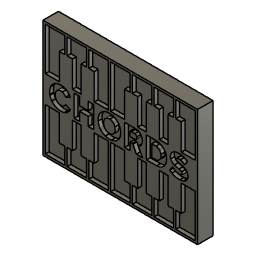
CHORDS Token (Autodesk Fusion 360 design; units mm, degrees)
Autodesk Fusion 360 part; units mm, degrees
(part 1 of 2)
sketch "Sketch1" plane through (0, 0, 0) normal (0, 0, 1) x (1, 0, 0)
  spline S0 degree 3 poles (0.0228, -10.5702) (0.0228, -7.0468) (0.0228, -3.5348) (0.0228, -0.0228) knots 0 0 0 0 1 1 1 1
  spline S1 degree 3 poles (0.0228, -0.0228) (13.3419, -0.0228) (26.6609, -0.0228) (39.98, -0.0228) knots 0 0 0 0 1 1 1 1
  spline S2 degree 3 poles (39.98, -0.0228) (39.98, -10.107) (39.98, -20.1912) (39.98, -30.2754) knots 0 0 0 0 1 1 1 1
  spline S3 degree 3 poles (39.98, -30.2754) (26.6609, -30.2754) (13.3419, -30.2754) (0.0228, -30.2754) knots 0 0 0 0 1 1 1 1
  spline S4 degree 3 poles (0.0228, -30.2754) (0.0228, -23.7108) (0.0228, -17.1462) (0.0228, -10.5702) knots 0 0 0 0 1 1 1 1
  spline S5 degree 3 poles (1.4466, -0.5923) (1.1634, -0.5923) (0.8802, -0.5923) (0.5988, -0.5923) knots 0 0 0 0 1 1 1 1
  spline S6 degree 3 poles (0.5988, -0.5923) (0.5988, -4.2974) (0.5988, -7.9893) (0.5988, -11.68) knots 0 0 0 0 1 1 1 1
  spline S7 degree 3 poles (0.5988, -11.68) (1.8142, -11.68) (3.0232, -11.68) (4.2411, -11.68) knots 0 0 0 0 1 1 1 1
  spline S8 degree 3 poles (4.2411, -11.68) (4.2411, -9.409) (4.2411, -7.1446) (4.2411, -4.8711) knots 0 0 0 0 1 1 1 1
  spline S9 degree 3 poles (4.2411, -4.8711) (4.715, -4.8711) (5.1799, -4.8711) (5.643, -4.8711) knots 0 0 0 0 1 1 1 1
  spline S10 degree 3 poles (5.643, -4.8711) (5.643, -3.4404) (5.643, -2.0188) (5.643, -0.5923) knots 0 0 0 0 1 1 1 1
  spline S11 degree 3 poles (5.643, -0.5923) (4.2474, -0.5923) (2.8584, -0.5923) (1.4466, -0.5923) knots 0 0 0 0 1 1 1 1
  spline S12 degree 3 poles (35.7656, -24.9334) (35.7656, -25.0951) (35.7656, -25.2569) (35.7656, -25.4274) knots 0 0 0 0 1 1 1 1
  spline S13 degree 3 poles (35.7656, -25.4274) (35.2876, -25.4274) (34.8227, -25.4274) (34.3599, -25.4274) knots 0 0 0 0 1 1 1 1
  spline S14 degree 3 poles (34.3599, -25.4274) (34.3599, -26.8581) (34.3599, -28.2796) (34.3599, -29.6993) knots 0 0 0 0 1 1 1 1
  spline S15 degree 3 poles (34.3599, -29.6993) (36.0463, -29.6993) (37.726, -29.6993) (39.4039, -29.6993) knots 0 0 0 0 1 1 1 1
  spline S16 degree 3 poles (39.4039, -29.6993) (39.4039, -26.0006) (39.4039, -22.3087) (39.4039, -18.6184) knots 0 0 0 0 1 1 1 1
  spline S17 degree 3 poles (39.4039, -18.6184) (38.1884, -18.6184) (36.9794, -18.6184) (35.7656, -18.6184) knots 0 0 0 0 1 1 1 1
  spline S18 degree 3 poles (35.7656, -18.6184) (35.7656, -20.7202) (35.7656, -22.8154) (35.7656, -24.9334) knots 0 0 0 0 1 1 1 1
  spline S19 degree 3 poles (18.0992, -18.6118) (17.8919, -18.6118) (17.6847, -18.6118) (17.4792, -18.6118) knots 0 0 0 0 1 1 1 1
  spline S20 degree 3 poles (17.4792, -18.6118) (17.4792, -22.3169) (17.4792, -26.0088) (17.4792, -29.6995) knots 0 0 0 0 1 1 1 1
  spline S21 degree 3 poles (17.4792, -29.6995) (19.1654, -29.6995) (20.8452, -29.6995) (22.5235, -29.6995) knots 0 0 0 0 1 1 1 1
  spline S22 degree 3 poles (22.5235, -29.6995) (22.5235, -28.2714) (22.5235, -26.8498) (22.5235, -25.4192) knots 0 0 0 0 1 1 1 1
  spline S23 degree 3 poles (22.5235, -25.4192) (22.0522, -25.4192) (21.5873, -25.4192) (21.1136, -25.4192) knots 0 0 0 0 1 1 1 1
  spline S24 degree 3 poles (21.1136, -25.4192) (21.1136, -23.1456) (21.1136, -20.8812) (21.1136, -18.6118) knots 0 0 0 0 1 1 1 1
  spline S25 degree 3 poles (21.1136, -18.6118) (20.1104, -18.6118) (19.1162, -18.6118) (18.0992, -18.6118) knots 0 0 0 0 1 1 1 1
  spline S26 degree 3 poles (13.2014, -29.7059) (14.4337, -29.7059) (15.6659, -29.7059) (16.8968, -29.7059) knots 0 0 0 0 1 1 1 1
  spline S27 degree 3 poles (16.8968, -29.7059) (16.8968, -26.0009) (16.8968, -22.309) (16.8968, -18.6182) knots 0 0 0 0 1 1 1 1
  spline S28 degree 3 poles (16.8968, -18.6182) (15.6814, -18.6182) (14.4725, -18.6182) (13.2545, -18.6182) knots 0 0 0 0 1 1 1 1
  spline S29 degree 3 poles (13.2545, -18.6182) (13.2545, -20.8891) (13.2545, -23.1535) (13.2545, -25.427) knots 0 0 0 0 1 1 1 1
  spline S30 degree 3 poles (13.2545, -25.427) (12.7807, -25.427) (12.3158, -25.427) (11.8524, -25.427) knots 0 0 0 0 1 1 1 1
  spline S31 degree 3 poles (11.8524, -25.427) (11.8524, -26.8577) (11.8524, -28.2793) (11.8524, -29.7059) knots 0 0 0 0 1 1 1 1
  spline S32 degree 3 poles (11.8524, -29.7059) (12.2988, -29.7059) (12.7387, -29.7059) (13.2014, -29.7059) knots 0 0 0 0 1 1 1 1
  spline S33 degree 3 poles (0.5923, -23.5438) (0.5923, -25.5961) (0.5923, -27.6485) (0.5923, -29.6995) knots 0 0 0 0 1 1 1 1
  spline S34 degree 3 poles (0.5923, -29.6995) (2.285, -29.6995) (3.9647, -29.6995) (5.6431, -29.6995) knots 0 0 0 0 1 1 1 1
  spline S35 degree 3 poles (5.6431, -29.6995) (5.6431, -28.2714) (5.6431, -26.8498) (5.6431, -25.4192) knots 0 0 0 0 1 1 1 1
  spline S36 degree 3 poles (5.6431, -25.4192) (5.1718, -25.4192) (4.7069, -25.4192) (4.2331, -25.4192) knots 0 0 0 0 1 1 1 1
  spline S37 degree 3 poles (4.2331, -25.4192) (4.2331, -23.1456) (4.2331, -20.8812) (4.2331, -18.6184) knots 0 0 0 0 1 1 1 1
  spline S38 degree 3 poles (4.2331, -18.6184) (3.0151, -18.6184) (1.8062, -18.6184) (0.5923, -18.6184) knots 0 0 0 0 1 1 1 1
  spline S39 degree 3 poles (0.5923, -18.6184) (0.5923, -20.2569) (0.5923, -21.889) (0.5923, -23.5438) knots 0 0 0 0 1 1 1 1
  spline S40 degree 3 poles (39.4105, -11.5811) (39.4105, -7.9193) (39.4105, -4.2574) (39.4105, -0.5998) knots 0 0 0 0 1 1 1 1
  spline S41 degree 3 poles (39.4105, -0.5998) (37.7158, -0.5998) (36.036, -0.5998) (34.3607, -0.5998) knots 0 0 0 0 1 1 1 1
  spline S42 degree 3 poles (34.3607, -0.5998) (34.3607, -2.0289) (34.3607, -3.4505) (34.3607, -4.8812) knots 0 0 0 0 1 1 1 1
  spline S43 degree 3 poles (34.3607, -4.8812) (34.8331, -4.8812) (35.2981, -4.8812) (35.7718, -4.8812) knots 0 0 0 0 1 1 1 1
  spline S44 degree 3 poles (35.7718, -4.8812) (35.7718, -7.1548) (35.7718, -9.4192) (35.7718, -11.6865) knots 0 0 0 0 1 1 1 1
  spline S45 degree 3 poles (35.7718, -11.6865) (36.9652, -11.6865) (38.1496, -11.6858) (39.3339, -11.6881) knots 0 0 0 0 1 1 1 1
  spline S46 degree 3 poles (39.3339, -11.6881) (39.4036, -11.6882) (39.4194, -11.6627) (39.4105, -11.5811) knots 0 0 0 0 1 1 1 1
  spline S47 degree 3 poles (16.9032, -10.2855) (16.9032, -7.0562) (16.9032, -3.8269) (16.9032, -0.5987) knots 0 0 0 0 1 1 1 1
  spline S48 degree 3 poles (16.9032, -0.5987) (15.2107, -0.5987) (13.5309, -0.5987) (11.8524, -0.5987) knots 0 0 0 0 1 1 1 1
  spline S49 degree 3 poles (11.8524, -0.5987) (11.8524, -2.0267) (11.8524, -3.4483) (11.8524, -4.8789) knots 0 0 0 0 1 1 1 1
  spline S50 degree 3 poles (11.8524, -4.8789) (12.3236, -4.8789) (12.7885, -4.8789) (13.2623, -4.8789) knots 0 0 0 0 1 1 1 1
  spline S51 degree 3 poles (13.2623, -4.8789) (13.2623, -7.1525) (13.2623, -9.4169) (13.2623, -11.6799) knots 0 0 0 0 1 1 1 1
  spline S52 degree 3 poles (13.2623, -11.6799) (14.4802, -11.6799) (15.6892, -11.6799) (16.9032, -11.6799) knots 0 0 0 0 1 1 1 1
  spline S53 degree 3 poles (16.9032, -11.6799) (16.9032, -11.2184) (16.9032, -10.7633) (16.9032, -10.2855) knots 0 0 0 0 1 1 1 1
  spline S54 degree 3 poles (21.1176, -8.1213) (21.1176, -7.0409) (21.1176, -5.9605) (21.1176, -4.871) knots 0 0 0 0 1 1 1 1
  spline S55 degree 3 poles (21.1176, -4.871) (21.5955, -4.871) (22.0604, -4.871) (22.5234, -4.871) knots 0 0 0 0 1 1 1 1
  spline S56 degree 3 poles (22.5234, -4.871) (22.5234, -3.4403) (22.5234, -2.0187) (22.5234, -0.5989) knots 0 0 0 0 1 1 1 1
  spline S57 degree 3 poles (22.5234, -0.5989) (20.8371, -0.5989) (19.1573, -0.5989) (17.4793, -0.5989) knots 0 0 0 0 1 1 1 1
  spline S58 degree 3 poles (17.4793, -0.5989) (17.4793, -4.2975) (17.4793, -7.9895) (17.4793, -11.6799) knots 0 0 0 0 1 1 1 1
  spline S59 degree 3 poles (17.4793, -11.6799) (18.6947, -11.6799) (19.9037, -11.6799) (21.1176, -11.6799) knots 0 0 0 0 1 1 1 1
  spline S60 degree 3 poles (21.1176, -11.6799) (21.1176, -10.4969) (21.1176, -9.3205) (21.1176, -8.1213) knots 0 0 0 0 1 1 1 1
  spline S61 degree 3 poles (11.2764, -0.6533) (11.2844, -0.5523) (11.2065, -0.5941) (11.1663, -0.5941) knots 0 0 0 0 1 1 1 1
  spline S62 degree 3 poles (11.1663, -0.5941) (9.549, -0.592) (7.9316, -0.5923) (6.3143, -0.5923) knots 0 0 0 0 1 1 1 1
  spline S63 degree 3 poles (6.3143, -0.5923) (6.2851, -0.5923) (6.2559, -0.5923) (6.2243, -0.5923) knots 0 0 0 0 1 1 1 1
  spline S64 degree 3 poles (6.2243, -0.5923) (6.2243, -2.0242) (6.2243, -3.4458) (6.2243, -4.8764) knots 0 0 0 0 1 1 1 1
  spline S65 degree 3 poles (6.2243, -4.8764) (6.6943, -4.8764) (7.1592, -4.8764) (7.633, -4.8764) knots 0 0 0 0 1 1 1 1
  spline S66 degree 3 poles (7.633, -4.8764) (7.633, -7.15) (7.633, -9.4144) (7.633, -11.6812) knots 0 0 0 0 1 1 1 1
  spline S67 degree 3 poles (7.633, -11.6812) (8.3802, -11.6812) (9.1183, -11.6812) (9.8655, -11.6812) knots 0 0 0 0 1 1 1 1
  spline S68 degree 3 poles (9.8655, -11.6812) (9.8655, -9.4115) (9.8655, -7.147) (9.8655, -4.8735) knots 0 0 0 0 1 1 1 1
  spline S69 degree 3 poles (9.8655, -4.8735) (10.3393, -4.8735) (10.8042, -4.8735) (11.2764, -4.8735) knots 0 0 0 0 1 1 1 1
  spline S70 degree 3 poles (11.2764, -4.8735) (11.2764, -3.4681) (11.2764, -2.0718) (11.2764, -0.6533) knots 0 0 0 0 1 1 1 1
  spline S71 degree 3 poles (30.5374, -29.7059) (31.6178, -29.7059) (32.6982, -29.7059) (33.7772, -29.7059) knots 0 0 0 0 1 1 1 1
  spline S72 degree 3 poles (33.7772, -29.7059) (33.7772, -28.2714) (33.7772, -26.8498) (33.7772, -25.4192) knots 0 0 0 0 1 1 1 1
  spline S73 degree 3 poles (33.7772, -25.4192) (33.3058, -25.4192) (32.8409, -25.4192) (32.3672, -25.4192) knots 0 0 0 0 1 1 1 1
  spline S74 degree 3 poles (32.3672, -25.4192) (32.3672, -23.1457) (32.3672, -20.8813) (32.3672, -18.6183) knots 0 0 0 0 1 1 1 1
  spline S75 degree 3 poles (32.3672, -18.6183) (31.6201, -18.6183) (30.8819, -18.6183) (30.1348, -18.6183) knots 0 0 0 0 1 1 1 1
  spline S76 degree 3 poles (30.1348, -18.6183) (30.1348, -20.8893) (30.1348, -23.1537) (30.1348, -25.4271) knots 0 0 0 0 1 1 1 1
  spline S77 degree 3 poles (30.1348, -25.4271) (29.661, -25.4271) (29.1961, -25.4271) (28.7329, -25.4271) knots 0 0 0 0 1 1 1 1
  spline S78 degree 3 poles (28.7329, -25.4271) (28.7329, -26.8578) (28.7329, -28.2794) (28.7329, -29.7059) knots 0 0 0 0 1 1 1 1
  spline S79 degree 3 poles (28.7329, -29.7059) (29.3312, -29.7059) (29.9229, -29.7059) (30.5374, -29.7059) knots 0 0 0 0 1 1 1 1
  spline S80 degree 3 poles (26.0952, -29.7059) (26.7808, -29.7059) (27.4663, -29.7059) (28.1503, -29.7059) knots 0 0 0 0 1 1 1 1
  spline S81 degree 3 poles (28.1503, -29.7059) (28.1503, -28.2713) (28.1503, -26.8497) (28.1503, -25.4191) knots 0 0 0 0 1 1 1 1
  spline S82 degree 3 poles (28.1503, -25.4191) (27.679, -25.4191) (27.2141, -25.4191) (26.7404, -25.4191) knots 0 0 0 0 1 1 1 1
  spline S83 degree 3 poles (26.7404, -25.4191) (26.7404, -23.1456) (26.7404, -20.8812) (26.7404, -18.6183) knots 0 0 0 0 1 1 1 1
  spline S84 degree 3 poles (26.7404, -18.6183) (25.9932, -18.6183) (25.255, -18.6183) (24.5079, -18.6183) knots 0 0 0 0 1 1 1 1
  spline S85 degree 3 poles (24.5079, -18.6183) (24.5079, -20.8893) (24.5079, -23.1537) (24.5079, -25.4272) knots 0 0 0 0 1 1 1 1
  spline S86 degree 3 poles (24.5079, -25.4272) (24.0341, -25.4272) (23.5692, -25.4272) (23.1061, -25.4272) knots 0 0 0 0 1 1 1 1
  spline S87 degree 3 poles (23.1061, -25.4272) (23.1061, -26.8579) (23.1061, -28.2794) (23.1061, -29.7059) knots 0 0 0 0 1 1 1 1
  spline S88 degree 3 poles (23.1061, -29.7059) (24.0993, -29.7059) (25.0858, -29.7059) (26.0952, -29.7059) knots 0 0 0 0 1 1 1 1
  spline S89 degree 3 poles (11.2764, -29.1478) (11.2764, -27.908) (11.2764, -26.6681) (11.2764, -25.4192) knots 0 0 0 0 1 1 1 1
  spline S90 degree 3 poles (11.2764, -25.4192) (10.7986, -25.4192) (10.3337, -25.4192) (9.86, -25.4192) knots 0 0 0 0 1 1 1 1
  spline S91 degree 3 poles (9.86, -25.4192) (9.86, -23.1457) (9.86, -20.8813) (9.86, -18.6183) knots 0 0 0 0 1 1 1 1
  spline S92 degree 3 poles (9.86, -18.6183) (9.1128, -18.6183) (8.3747, -18.6183) (7.6276, -18.6183) knots 0 0 0 0 1 1 1 1
  spline S93 degree 3 poles (7.6276, -18.6183) (7.6276, -20.8892) (7.6276, -23.1536) (7.6276, -25.4271) knots 0 0 0 0 1 1 1 1
  spline S94 degree 3 poles (7.6276, -25.4271) (7.1538, -25.4271) (6.6889, -25.4271) (6.2256, -25.4271) knots 0 0 0 0 1 1 1 1
  spline S95 degree 3 poles (6.2256, -25.4271) (6.2256, -26.8578) (6.2256, -28.2793) (6.2256, -29.6994) knots 0 0 0 0 1 1 1 1
  spline S96 degree 3 poles (6.2256, -29.6994) (7.9119, -29.6994) (9.5916, -29.6994) (11.2764, -29.6994) knots 0 0 0 0 1 1 1 1
  spline S97 degree 3 poles (11.2764, -29.6994) (11.2764, -29.5188) (11.2764, -29.3447) (11.2764, -29.1478) knots 0 0 0 0 1 1 1 1
  spline S98 degree 3 poles (30.1388, -7.9618) (30.1388, -9.2017) (30.1388, -10.4415) (30.1388, -11.6799) knots 0 0 0 0 1 1 1 1
  spline S99 degree 3 poles (30.1388, -11.6799) (30.8899, -11.6799) (31.6281, -11.6799) (32.3752, -11.6799) knots 0 0 0 0 1 1 1 1
  spline S100 degree 3 poles (32.3752, -11.6799) (32.3752, -9.409) (32.3752, -7.1446) (32.3752, -4.8711) knots 0 0 0 0 1 1 1 1
  spline S101 degree 3 poles (32.3752, -4.8711) (32.849, -4.8711) (33.3139, -4.8711) (33.7771, -4.8711) knots 0 0 0 0 1 1 1 1
  spline S102 degree 3 poles (33.7771, -4.8711) (33.7771, -3.4404) (33.7771, -2.0189) (33.7771, -0.5988) knots 0 0 0 0 1 1 1 1
  spline S103 degree 3 poles (33.7771, -0.5988) (32.0909, -0.5988) (30.4112, -0.5988) (28.7329, -0.5988) knots 0 0 0 0 1 1 1 1
  spline S104 degree 3 poles (28.7329, -0.5988) (28.7329, -2.0269) (28.7329, -3.4484) (28.7329, -4.8791) knots 0 0 0 0 1 1 1 1
  spline S105 degree 3 poles (28.7329, -4.8791) (29.2042, -4.8791) (29.6691, -4.8791) (30.1388, -4.8791) knots 0 0 0 0 1 1 1 1
  spline S106 degree 3 poles (30.1388, -4.8791) (30.1388, -5.9051) (30.1388, -6.9221) (30.1388, -7.9618) knots 0 0 0 0 1 1 1 1
  spline S107 degree 3 poles (26.7445, -9.4198) (26.7445, -7.9066) (26.7445, -6.3934) (26.7445, -4.8711) knots 0 0 0 0 1 1 1 1
  spline S108 degree 3 poles (26.7445, -4.8711) (27.2222, -4.8711) (27.6871, -4.8711) (28.1503, -4.8711) knots 0 0 0 0 1 1 1 1
  spline S109 degree 3 poles (28.1503, -4.8711) (28.1503, -3.4404) (28.1503, -2.0189) (28.1503, -0.5988) knots 0 0 0 0 1 1 1 1
  spline S110 degree 3 poles (28.1503, -0.5988) (26.4641, -0.5988) (24.7843, -0.5988) (23.1061, -0.5988) knots 0 0 0 0 1 1 1 1
  spline S111 degree 3 poles (23.1061, -0.5988) (23.1061, -2.0269) (23.1061, -3.4484) (23.1061, -4.8791) knots 0 0 0 0 1 1 1 1
  spline S112 degree 3 poles (23.1061, -4.8791) (23.5774, -4.8791) (24.0423, -4.8791) (24.516, -4.8791) knots 0 0 0 0 1 1 1 1
  spline S113 degree 3 poles (24.516, -4.8791) (24.516, -7.1526) (24.516, -9.417) (24.516, -11.6799) knots 0 0 0 0 1 1 1 1
  spline S114 degree 3 poles (24.516, -11.6799) (25.2631, -11.6799) (26.0013, -11.6799) (26.7445, -11.6799) knots 0 0 0 0 1 1 1 1
  spline S115 degree 3 poles (26.7445, -11.6799) (26.7445, -10.9298) (26.7445, -10.1862) (26.7445, -9.4198) knots 0 0 0 0 1 1 1 1
  spline S116 degree 3 poles (31.2674, -17.0863) (31.401, -16.8984) (31.5593, -16.7233) (31.6638, -16.5205) knots 0 0 0 0 1 1 1 1
  spline S117 degree 3 poles (31.6638, -16.5205) (32.0308, -15.8079) (32.0758, -15.0551) (31.8752, -14.2875) knots 0 0 0 0 1 1 1 1
  spline S118 degree 3 poles (31.8752, -14.2875) (31.68, -13.5405) (31.2249, -12.9974) (30.5351, -12.6532) knots 0 0 0 0 1 1 1 1
  spline S119 degree 3 poles (30.5351, -12.6532) (30.0644, -12.4183) (29.5596, -12.329) (29.0381, -12.3269) knots 0 0 0 0 1 1 1 1
  spline S120 degree 3 poles (29.0381, -12.3269) (28.3054, -12.3239) (27.5727, -12.3261) (26.8399, -12.3261) knots 0 0 0 0 1 1 1 1
  spline S121 degree 3 poles (26.8399, -12.3261) (26.8108, -12.3261) (26.7817, -12.3261) (26.7518, -12.3261) knots 0 0 0 0 1 1 1 1
  spline S122 degree 3 poles (26.7518, -12.3261) (26.7518, -14.2063) (26.7518, -16.0754) (26.7518, -17.9291) knots 0 0 0 0 1 1 1 1
  spline S123 degree 3 poles (26.7518, -17.9291) (27.6506, -17.9291) (28.5433, -17.9582) (29.4331, -17.9199) knots 0 0 0 0 1 1 1 1
  spline S124 degree 3 poles (29.4331, -17.9199) (30.1342, -17.8896) (30.7554, -17.6092) (31.2674, -17.0863) knots 0 0 0 0 1 1 1 1
  spline S125 degree 3 poles (25.0567, -12.7014) (24.6935, -12.4266) (24.2757, -12.3262) (23.8296, -12.325) knots 0 0 0 0 1 1 1 1
  spline S126 degree 3 poles (23.8296, -12.325) (22.9565, -12.3226) (22.0835, -12.3243) (21.2104, -12.3245) knots 0 0 0 0 1 1 1 1
  spline S127 degree 3 poles (21.2104, -12.3245) (21.1813, -12.3245) (21.1523, -12.327) (21.1233, -12.3284) knots 0 0 0 0 1 1 1 1
  spline S128 degree 3 poles (21.1233, -12.3284) (21.1233, -14.2057) (21.1233, -16.0751) (21.1233, -17.9455) knots 0 0 0 0 1 1 1 1
  spline S129 degree 3 poles (21.1233, -17.9455) (21.5938, -17.9455) (22.0586, -17.9455) (22.5324, -17.9455) knots 0 0 0 0 1 1 1 1
  spline S130 degree 3 poles (22.5324, -17.9455) (22.5324, -17.308) (22.5324, -16.6761) (22.5324, -16.0376) knots 0 0 0 0 1 1 1 1
  spline S131 degree 3 poles (22.5324, -16.0376) (22.7418, -16.0376) (22.9424, -16.0425) (23.1426, -16.0352) knots 0 0 0 0 1 1 1 1
  spline S132 degree 3 poles (23.1426, -16.0352) (23.2246, -16.0322) (23.2595, -16.0634) (23.2923, -16.1331) knots 0 0 0 0 1 1 1 1
  spline S133 degree 3 poles (23.2923, -16.1331) (23.5772, -16.739) (23.866, -17.3431) (24.1535, -17.9475) knots 0 0 0 0 1 1 1 1
  spline S134 degree 3 poles (24.1535, -17.9475) (24.6869, -17.9475) (25.2172, -17.9475) (25.7624, -17.9475) knots 0 0 0 0 1 1 1 1
  spline S135 degree 3 poles (25.7624, -17.9475) (25.39, -17.2541) (25.0223, -16.5698) (24.6542, -15.8845) knots 0 0 0 0 1 1 1 1
  spline S136 degree 3 poles (24.6542, -15.8845) (26.0292, -15.3556) (26.0221, -13.4204) (25.0567, -12.7014) knots 0 0 0 0 1 1 1 1
  spline S137 degree 3 poles (16.1529, -17.8935) (16.6625, -18.0645) (17.1838, -18.1067) (17.713, -18.02) knots 0 0 0 0 1 1 1 1
  spline S138 degree 3 poles (17.713, -18.02) (18.5444, -17.8837) (19.2139, -17.4852) (19.6675, -16.7638) knots 0 0 0 0 1 1 1 1
  spline S139 degree 3 poles (19.6675, -16.7638) (20.0864, -16.0975) (20.1938, -15.3643) (20.0663, -14.5989) knots 0 0 0 0 1 1 1 1
  spline S140 degree 3 poles (20.0663, -14.5989) (19.9233, -13.7403) (19.4853, -13.068) (18.7243, -12.6285) knots 0 0 0 0 1 1 1 1
  spline S141 degree 3 poles (18.7243, -12.6285) (18.1513, -12.2977) (17.5266, -12.1895) (16.8716, -12.2536) knots 0 0 0 0 1 1 1 1
  spline S142 degree 3 poles (16.8716, -12.2536) (16.0569, -12.3333) (15.3695, -12.6649) (14.8619, -13.3182) knots 0 0 0 0 1 1 1 1
  spline S143 degree 3 poles (14.8619, -13.3182) (14.3755, -13.9444) (14.2022, -14.6676) (14.2807, -15.4476) knots 0 0 0 0 1 1 1 1
  spline S144 degree 3 poles (14.2807, -15.4476) (14.4002, -16.6354) (15.0088, -17.4609) (16.1529, -17.8935) knots 0 0 0 0 1 1 1 1
  spline S145 degree 3 poles (10.6272, -14.4201) (10.2378, -14.4201) (9.8484, -14.4201) (9.4503, -14.4201) knots 0 0 0 0 1 1 1 1
  spline S146 degree 3 poles (9.4503, -14.4201) (9.4503, -13.7148) (9.4503, -13.0222) (9.4503, -12.3306) knots 0 0 0 0 1 1 1 1
  spline S147 degree 3 poles (9.4503, -12.3306) (8.9766, -12.3306) (8.5119, -12.3306) (8.0472, -12.3306) knots 0 0 0 0 1 1 1 1
  spline S148 degree 3 poles (8.0472, -12.3306) (8.0472, -14.206) (8.0472, -16.0752) (8.0472, -17.9455) knots 0 0 0 0 1 1 1 1
  spline S149 degree 3 poles (8.0472, -17.9455) (8.5177, -17.9455) (8.9824, -17.9455) (9.4552, -17.9455) knots 0 0 0 0 1 1 1 1
  spline S150 degree 3 poles (9.4552, -17.9455) (9.4552, -17.1901) (9.4552, -16.4402) (9.4552, -15.6849) knots 0 0 0 0 1 1 1 1
  spline S151 degree 3 poles (9.4552, -15.6849) (10.2088, -15.6849) (10.9543, -15.6849) (11.712, -15.6849) knots 0 0 0 0 1 1 1 1
  spline S152 degree 3 poles (11.712, -15.6849) (11.712, -16.4429) (11.712, -17.1955) (11.712, -17.9437) knots 0 0 0 0 1 1 1 1
  spline S153 degree 3 poles (11.712, -17.9437) (12.1889, -17.9437) (12.6537, -17.9437) (13.1148, -17.9437) knots 0 0 0 0 1 1 1 1
  spline S154 degree 3 poles (13.1148, -17.9437) (13.1148, -16.0672) (13.1148, -14.198) (13.1148, -12.3311) knots 0 0 0 0 1 1 1 1
  spline S155 degree 3 poles (13.1148, -12.3311) (12.6432, -12.3311) (12.1785, -12.3311) (11.7049, -12.3311) knots 0 0 0 0 1 1 1 1
  spline S156 degree 3 poles (11.7049, -12.3311) (11.7049, -13.0303) (11.7049, -13.7229) (11.7049, -14.4201) knots 0 0 0 0 1 1 1 1
  spline S157 degree 3 poles (11.7049, -14.4201) (11.3473, -14.4201) (10.9986, -14.4201) (10.6272, -14.4201) knots 0 0 0 0 1 1 1 1
  spline S158 degree 3 poles (35.429, -18.0595) (35.7152, -18.0078) (36.0122, -17.9886) (36.2859, -17.8987) knots 0 0 0 0 1 1 1 1
  spline S159 degree 3 poles (36.2859, -17.8987) (37.453, -17.5153) (37.6514, -16.4372) (37.4532, -15.7221) knots 0 0 0 0 1 1 1 1
  spline S160 degree 3 poles (37.4532, -15.7221) (37.3295, -15.2758) (37.0095, -15.0019) (36.6092, -14.8078) knots 0 0 0 0 1 1 1 1
  spline S161 degree 3 poles (36.6092, -14.8078) (36.1929, -14.6061) (35.7418, -14.5212) (35.2961, -14.416) knots 0 0 0 0 1 1 1 1
  spline S162 degree 3 poles (35.2961, -14.416) (35.0655, -14.3616) (34.8301, -14.3042) (34.6169, -14.2051) knots 0 0 0 0 1 1 1 1
  spline S163 degree 3 poles (34.6169, -14.2051) (34.3613, -14.0864) (34.3582, -13.7521) (34.5927, -13.5913) knots 0 0 0 0 1 1 1 1
  spline S164 degree 3 poles (34.5927, -13.5913) (34.6447, -13.5556) (34.7061, -13.5289) (34.7671, -13.5119) knots 0 0 0 0 1 1 1 1
  spline S165 degree 3 poles (34.7671, -13.5119) (35.019, -13.4418) (35.2713, -13.4707) (35.5216, -13.5236) knots 0 0 0 0 1 1 1 1
  spline S166 degree 3 poles (35.5216, -13.5236) (35.9294, -13.6098) (36.2925, -13.7907) (36.6186, -14.0557) knots 0 0 0 0 1 1 1 1
  spline S167 degree 3 poles (36.6186, -14.0557) (36.8759, -13.7079) (37.1302, -13.3644) (37.3871, -13.0172) knots 0 0 0 0 1 1 1 1
  spline S168 degree 3 poles (37.3871, -13.0172) (37.3229, -12.9656) (37.2652, -12.9163) (37.2046, -12.8709) knots 0 0 0 0 1 1 1 1
  spline S169 degree 3 poles (37.2046, -12.8709) (36.6315, -12.4423) (35.9773, -12.2575) (35.2711, -12.2358) knots 0 0 0 0 1 1 1 1
  spline S170 degree 3 poles (35.2711, -12.2358) (34.8576, -12.223) (34.4539, -12.2782) (34.0699, -12.4405) knots 0 0 0 0 1 1 1 1
  spline S171 degree 3 poles (34.0699, -12.4405) (33.2042, -12.8062) (32.7844, -13.6938) (33.074, -14.5448) knots 0 0 0 0 1 1 1 1
  spline S172 degree 3 poles (33.074, -14.5448) (33.2291, -15.0004) (33.5664, -15.2834) (33.9981, -15.4393) knots 0 0 0 0 1 1 1 1
  spline S173 degree 3 poles (33.9981, -15.4393) (34.3771, -15.5761) (34.7748, -15.6619) (35.1656, -15.765) knots 0 0 0 0 1 1 1 1
  spline S174 degree 3 poles (35.1656, -15.765) (35.4179, -15.8315) (35.6796, -15.8714) (35.9019, -16.0198) knots 0 0 0 0 1 1 1 1
  spline S175 degree 3 poles (35.9019, -16.0198) (36.1425, -16.1803) (36.1534, -16.4769) (35.9212, -16.649) knots 0 0 0 0 1 1 1 1
  spline S176 degree 3 poles (35.9212, -16.649) (35.8382, -16.7105) (35.7366, -16.7547) (35.6367, -16.784) knots 0 0 0 0 1 1 1 1
  spline S177 degree 3 poles (35.6367, -16.784) (35.4142, -16.8493) (35.1855, -16.8335) (34.9593, -16.8) knots 0 0 0 0 1 1 1 1
  spline S178 degree 3 poles (34.9593, -16.8) (34.416, -16.7195) (33.9548, -16.4754) (33.5594, -16.0811) knots 0 0 0 0 1 1 1 1
  spline S179 degree 3 poles (33.5594, -16.0811) (33.312, -16.4435) (33.0667, -16.8029) (32.8062, -17.1844) knots 0 0 0 0 1 1 1 1
  spline S180 degree 3 poles (32.8062, -17.1844) (32.9868, -17.3185) (33.1571, -17.4644) (33.3454, -17.5812) knots 0 0 0 0 1 1 1 1
  spline S181 degree 3 poles (33.3454, -17.5812) (33.9769, -17.9731) (34.6784, -18.0797) (35.429, -18.0595) knots 0 0 0 0 1 1 1 1
  spline S182 degree 3 poles (1.7635, -15.742) (1.8461, -16.1886) (2.0179, -16.5963) (2.2925, -16.9597) knots 0 0 0 0 1 1 1 1
  spline S183 degree 3 poles (2.2925, -16.9597) (3.0452, -17.956) (4.3949, -18.2671) (5.4961, -17.9369) knots 0 0 0 0 1 1 1 1
  spline S184 degree 3 poles (5.4961, -17.9369) (6.2227, -17.719) (6.7147, -17.2311) (7.0532, -16.5552) knots 0 0 0 0 1 1 1 1
  spline S185 degree 3 poles (7.0532, -16.5552) (6.6455, -16.3561) (6.2462, -16.1611) (5.8469, -15.9661) knots 0 0 0 0 1 1 1 1
  spline S186 degree 3 poles (5.8469, -15.9661) (5.6028, -16.4677) (5.2156, -16.7636) (4.6612, -16.7813) knots 0 0 0 0 1 1 1 1
  spline S187 degree 3 poles (4.6612, -16.7813) (4.104, -16.799) (3.665, -16.5497) (3.3893, -16.0671) knots 0 0 0 0 1 1 1 1
  spline S188 degree 3 poles (3.3893, -16.0671) (3.0431, -15.461) (3.0448, -14.8341) (3.3907, -14.2271) knots 0 0 0 0 1 1 1 1
  spline S189 degree 3 poles (3.3907, -14.2271) (3.7265, -13.6377) (4.4189, -13.3734) (5.0331, -13.581) knots 0 0 0 0 1 1 1 1
  spline S190 degree 3 poles (5.0331, -13.581) (5.4119, -13.709) (5.6784, -13.9656) (5.8446, -14.3334) knots 0 0 0 0 1 1 1 1
  spline S191 degree 3 poles (5.8446, -14.3334) (6.2483, -14.1361) (6.6476, -13.9409) (7.0529, -13.7428) knots 0 0 0 0 1 1 1 1
  spline S192 degree 3 poles (7.0529, -13.7428) (6.7834, -13.1999) (6.4138, -12.7708) (5.874, -12.507) knots 0 0 0 0 1 1 1 1
  spline S193 degree 3 poles (5.874, -12.507) (5.3126, -12.2327) (4.7174, -12.1777) (4.1098, -12.2797) knots 0 0 0 0 1 1 1 1
  spline S194 degree 3 poles (4.1098, -12.2797) (3.1324, -12.4438) (2.4019, -12.9553) (1.9794, -13.8657) knots 0 0 0 0 1 1 1 1
  spline S195 degree 3 poles (1.9794, -13.8657) (1.7044, -14.4582) (1.6566, -15.083) (1.7635, -15.742) knots 0 0 0 0 1 1 1 1
  spline S196 degree 3 poles (1.458, -0.5923) (2.8584, -0.5923) (4.2474, -0.5923) (5.643, -0.5923) knots 0 0 0 0 1 1 1 1
  spline S197 degree 3 poles (5.643, -0.5923) (5.643, -2.0188) (5.643, -3.4404) (5.643, -4.8711) knots 0 0 0 0 1 1 1 1
  spline S198 degree 3 poles (5.643, -4.8711) (5.1799, -4.8711) (4.715, -4.8711) (4.2411, -4.8711) knots 0 0 0 0 1 1 1 1
  spline S199 degree 3 poles (4.2411, -4.8711) (4.2411, -7.1446) (4.2411, -9.409) (4.2411, -11.68) knots 0 0 0 0 1 1 1 1
  spline S200 degree 3 poles (4.2411, -11.68) (3.0232, -11.68) (1.8142, -11.68) (0.5988, -11.68) knots 0 0 0 0 1 1 1 1
  spline S201 degree 3 poles (0.5988, -11.68) (0.5988, -7.9893) (0.5988, -4.2974) (0.5988, -0.5923) knots 0 0 0 0 1 1 1 1
  spline S202 degree 3 poles (0.5988, -0.5923) (0.8802, -0.5923) (1.1634, -0.5923) (1.458, -0.5923) knots 0 0 0 0 1 1 1 1
  spline S203 degree 3 poles (35.7656, -24.922) (35.7656, -22.8154) (35.7656, -20.7202) (35.7656, -18.6184) knots 0 0 0 0 1 1 1 1
  spline S204 degree 3 poles (35.7656, -18.6184) (36.9794, -18.6184) (38.1884, -18.6184) (39.4039, -18.6184) knots 0 0 0 0 1 1 1 1
  spline S205 degree 3 poles (39.4039, -18.6184) (39.4039, -22.3087) (39.4039, -26.0006) (39.4039, -29.6993) knots 0 0 0 0 1 1 1 1
  spline S206 degree 3 poles (39.4039, -29.6993) (37.726, -29.6993) (36.0463, -29.6993) (34.3599, -29.6993) knots 0 0 0 0 1 1 1 1
  spline S207 degree 3 poles (34.3599, -29.6993) (34.3599, -28.2796) (34.3599, -26.8581) (34.3599, -25.4274) knots 0 0 0 0 1 1 1 1
  spline S208 degree 3 poles (34.3599, -25.4274) (34.8227, -25.4274) (35.2876, -25.4274) (35.7656, -25.4274) knots 0 0 0 0 1 1 1 1
  spline S209 degree 3 poles (35.7656, -25.4274) (35.7656, -25.2569) (35.7656, -25.0951) (35.7656, -24.922) knots 0 0 0 0 1 1 1 1
  spline S210 degree 3 poles (18.1106, -18.6118) (19.1162, -18.6118) (20.1104, -18.6118) (21.1136, -18.6118) knots 0 0 0 0 1 1 1 1
  spline S211 degree 3 poles (21.1136, -18.6118) (21.1136, -20.8812) (21.1136, -23.1456) (21.1136, -25.4192) knots 0 0 0 0 1 1 1 1
  spline S212 degree 3 poles (21.1136, -25.4192) (21.5873, -25.4192) (22.0522, -25.4192) (22.5235, -25.4192) knots 0 0 0 0 1 1 1 1
  spline S213 degree 3 poles (22.5235, -25.4192) (22.5235, -26.8498) (22.5235, -28.2714) (22.5235, -29.6995) knots 0 0 0 0 1 1 1 1
  spline S214 degree 3 poles (22.5235, -29.6995) (20.8452, -29.6995) (19.1654, -29.6995) (17.4792, -29.6995) knots 0 0 0 0 1 1 1 1
  spline S215 degree 3 poles (17.4792, -29.6995) (17.4792, -26.0088) (17.4792, -22.3169) (17.4792, -18.6118) knots 0 0 0 0 1 1 1 1
  spline S216 degree 3 poles (17.4792, -18.6118) (17.6847, -18.6118) (17.8919, -18.6118) (18.1106, -18.6118) knots 0 0 0 0 1 1 1 1
  spline S217 degree 3 poles (13.19, -29.7059) (12.7387, -29.7059) (12.2988, -29.7059) (11.8524, -29.7059) knots 0 0 0 0 1 1 1 1
  spline S218 degree 3 poles (11.8524, -29.7059) (11.8524, -28.2793) (11.8524, -26.8577) (11.8524, -25.427) knots 0 0 0 0 1 1 1 1
  spline S219 degree 3 poles (11.8524, -25.427) (12.3158, -25.427) (12.7807, -25.427) (13.2545, -25.427) knots 0 0 0 0 1 1 1 1
  spline S220 degree 3 poles (13.2545, -25.427) (13.2545, -23.1535) (13.2545, -20.8891) (13.2545, -18.6182) knots 0 0 0 0 1 1 1 1
  spline S221 degree 3 poles (13.2545, -18.6182) (14.4725, -18.6182) (15.6814, -18.6182) (16.8968, -18.6182) knots 0 0 0 0 1 1 1 1
  spline S222 degree 3 poles (16.8968, -18.6182) (16.8968, -22.309) (16.8968, -26.0009) (16.8968, -29.7059) knots 0 0 0 0 1 1 1 1
  spline S223 degree 3 poles (16.8968, -29.7059) (15.6659, -29.7059) (14.4337, -29.7059) (13.19, -29.7059) knots 0 0 0 0 1 1 1 1
  spline S224 degree 3 poles (0.5923, -23.5324) (0.5923, -21.889) (0.5923, -20.2569) (0.5923, -18.6184) knots 0 0 0 0 1 1 1 1
  spline S225 degree 3 poles (0.5923, -18.6184) (1.8062, -18.6184) (3.0151, -18.6184) (4.2331, -18.6184) knots 0 0 0 0 1 1 1 1
  spline S226 degree 3 poles (4.2331, -18.6184) (4.2331, -20.8812) (4.2331, -23.1456) (4.2331, -25.4192) knots 0 0 0 0 1 1 1 1
  spline S227 degree 3 poles (4.2331, -25.4192) (4.7069, -25.4192) (5.1718, -25.4192) (5.6431, -25.4192) knots 0 0 0 0 1 1 1 1
  spline S228 degree 3 poles (5.6431, -25.4192) (5.6431, -26.8498) (5.6431, -28.2714) (5.6431, -29.6995) knots 0 0 0 0 1 1 1 1
  spline S229 degree 3 poles (5.6431, -29.6995) (3.9647, -29.6995) (2.285, -29.6995) (0.5923, -29.6995) knots 0 0 0 0 1 1 1 1
  spline S230 degree 3 poles (0.5923, -29.6995) (0.5923, -27.6485) (0.5923, -25.5961) (0.5923, -23.5324) knots 0 0 0 0 1 1 1 1
  spline S231 degree 3 poles (39.4105, -11.5922) (39.4194, -11.6627) (39.4036, -11.6882) (39.3339, -11.6881) knots 0 0 0 0 1 1 1 1
  spline S232 degree 3 poles (39.3339, -11.6881) (38.1496, -11.6858) (36.9652, -11.6865) (35.7718, -11.6865) knots 0 0 0 0 1 1 1 1
  spline S233 degree 3 poles (35.7718, -11.6865) (35.7718, -9.4192) (35.7718, -7.1548) (35.7718, -4.8812) knots 0 0 0 0 1 1 1 1
  spline S234 degree 3 poles (35.7718, -4.8812) (35.2981, -4.8812) (34.8331, -4.8812) (34.3607, -4.8812) knots 0 0 0 0 1 1 1 1
  spline S235 degree 3 poles (34.3607, -4.8812) (34.3607, -3.4505) (34.3607, -2.0289) (34.3607, -0.5998) knots 0 0 0 0 1 1 1 1
  spline S236 degree 3 poles (34.3607, -0.5998) (36.036, -0.5998) (37.7158, -0.5998) (39.4105, -0.5998) knots 0 0 0 0 1 1 1 1
  spline S237 degree 3 poles (39.4105, -0.5998) (39.4105, -4.2574) (39.4105, -7.9193) (39.4105, -11.5922) knots 0 0 0 0 1 1 1 1
  spline S238 degree 3 poles (16.9032, -10.2968) (16.9032, -10.7633) (16.9032, -11.2184) (16.9032, -11.6799) knots 0 0 0 0 1 1 1 1
  spline S239 degree 3 poles (16.9032, -11.6799) (15.6892, -11.6799) (14.4802, -11.6799) (13.2623, -11.6799) knots 0 0 0 0 1 1 1 1
  spline S240 degree 3 poles (13.2623, -11.6799) (13.2623, -9.4169) (13.2623, -7.1525) (13.2623, -4.8789) knots 0 0 0 0 1 1 1 1
  spline S241 degree 3 poles (13.2623, -4.8789) (12.7885, -4.8789) (12.3236, -4.8789) (11.8524, -4.8789) knots 0 0 0 0 1 1 1 1
  spline S242 degree 3 poles (11.8524, -4.8789) (11.8524, -3.4483) (11.8524, -2.0267) (11.8524, -0.5987) knots 0 0 0 0 1 1 1 1
  spline S243 degree 3 poles (11.8524, -0.5987) (13.5309, -0.5987) (15.2107, -0.5987) (16.9032, -0.5987) knots 0 0 0 0 1 1 1 1
  spline S244 degree 3 poles (16.9032, -0.5987) (16.9032, -3.8269) (16.9032, -7.0562) (16.9032, -10.2968) knots 0 0 0 0 1 1 1 1
  spline S245 degree 3 poles (21.1176, -8.1327) (21.1176, -9.3205) (21.1176, -10.4969) (21.1176, -11.6799) knots 0 0 0 0 1 1 1 1
  spline S246 degree 3 poles (21.1176, -11.6799) (19.9037, -11.6799) (18.6947, -11.6799) (17.4793, -11.6799) knots 0 0 0 0 1 1 1 1
  spline S247 degree 3 poles (17.4793, -11.6799) (17.4793, -7.9895) (17.4793, -4.2975) (17.4793, -0.5989) knots 0 0 0 0 1 1 1 1
  spline S248 degree 3 poles (17.4793, -0.5989) (19.1573, -0.5989) (20.8371, -0.5989) (22.5234, -0.5989) knots 0 0 0 0 1 1 1 1
  spline S249 degree 3 poles (22.5234, -0.5989) (22.5234, -2.0187) (22.5234, -3.4403) (22.5234, -4.871) knots 0 0 0 0 1 1 1 1
  spline S250 degree 3 poles (22.5234, -4.871) (22.0604, -4.871) (21.5955, -4.871) (21.1176, -4.871) knots 0 0 0 0 1 1 1 1
  spline S251 degree 3 poles (21.1176, -4.871) (21.1176, -5.9605) (21.1176, -7.0409) (21.1176, -8.1327) knots 0 0 0 0 1 1 1 1
  spline S252 degree 3 poles (11.2764, -0.6644) (11.2764, -2.0718) (11.2764, -3.4681) (11.2764, -4.8735) knots 0 0 0 0 1 1 1 1
  spline S253 degree 3 poles (11.2764, -4.8735) (10.8042, -4.8735) (10.3393, -4.8735) (9.8655, -4.8735) knots 0 0 0 0 1 1 1 1
  spline S254 degree 3 poles (9.8655, -4.8735) (9.8655, -7.147) (9.8655, -9.4115) (9.8655, -11.6812) knots 0 0 0 0 1 1 1 1
  spline S255 degree 3 poles (9.8655, -11.6812) (9.1183, -11.6812) (8.3802, -11.6812) (7.633, -11.6812) knots 0 0 0 0 1 1 1 1
  spline S256 degree 3 poles (7.633, -11.6812) (7.633, -9.4144) (7.633, -7.15) (7.633, -4.8764) knots 0 0 0 0 1 1 1 1
  spline S257 degree 3 poles (7.633, -4.8764) (7.1592, -4.8764) (6.6943, -4.8764) (6.2243, -4.8764) knots 0 0 0 0 1 1 1 1
  spline S258 degree 3 poles (6.2243, -4.8764) (6.2243, -3.4458) (6.2243, -2.0242) (6.2243, -0.5923) knots 0 0 0 0 1 1 1 1
  spline S259 degree 3 poles (6.2243, -0.5923) (6.2559, -0.5923) (6.2851, -0.5923) (6.3143, -0.5923) knots 0 0 0 0 1 1 1 1
  spline S260 degree 3 poles (6.3143, -0.5923) (7.9316, -0.5923) (9.549, -0.592) (11.1663, -0.5941) knots 0 0 0 0 1 1 1 1
  spline S261 degree 3 poles (11.1663, -0.5941) (11.2065, -0.5941) (11.2844, -0.5523) (11.2764, -0.6644) knots 0 0 0 0 1 1 1 1
  spline S262 degree 3 poles (30.526, -29.7059) (29.9229, -29.7059) (29.3312, -29.7059) (28.7329, -29.7059) knots 0 0 0 0 1 1 1 1
  spline S263 degree 3 poles (28.7329, -29.7059) (28.7329, -28.2794) (28.7329, -26.8578) (28.7329, -25.4271) knots 0 0 0 0 1 1 1 1
  spline S264 degree 3 poles (28.7329, -25.4271) (29.1961, -25.4271) (29.661, -25.4271) (30.1348, -25.4271) knots 0 0 0 0 1 1 1 1
  spline S265 degree 3 poles (30.1348, -25.4271) (30.1348, -23.1537) (30.1348, -20.8893) (30.1348, -18.6183) knots 0 0 0 0 1 1 1 1
  spline S266 degree 3 poles (30.1348, -18.6183) (30.8819, -18.6183) (31.6201, -18.6183) (32.3672, -18.6183) knots 0 0 0 0 1 1 1 1
  spline S267 degree 3 poles (32.3672, -18.6183) (32.3672, -20.8813) (32.3672, -23.1457) (32.3672, -25.4192) knots 0 0 0 0 1 1 1 1
  spline S268 degree 3 poles (32.3672, -25.4192) (32.8409, -25.4192) (33.3058, -25.4192) (33.7772, -25.4192) knots 0 0 0 0 1 1 1 1
  spline S269 degree 3 poles (33.7772, -25.4192) (33.7772, -26.8498) (33.7772, -28.2714) (33.7772, -29.7059) knots 0 0 0 0 1 1 1 1
  spline S270 degree 3 poles (33.7772, -29.7059) (32.6982, -29.7059) (31.6178, -29.7059) (30.526, -29.7059) knots 0 0 0 0 1 1 1 1
  spline S271 degree 3 poles (26.0838, -29.7059) (25.0858, -29.7059) (24.0993, -29.7059) (23.1061, -29.7059) knots 0 0 0 0 1 1 1 1
  spline S272 degree 3 poles (23.1061, -29.7059) (23.1061, -28.2794) (23.1061, -26.8579) (23.1061, -25.4272) knots 0 0 0 0 1 1 1 1
  spline S273 degree 3 poles (23.1061, -25.4272) (23.5692, -25.4272) (24.0341, -25.4272) (24.5079, -25.4272) knots 0 0 0 0 1 1 1 1
  spline S274 degree 3 poles (24.5079, -25.4272) (24.5079, -23.1537) (24.5079, -20.8893) (24.5079, -18.6183) knots 0 0 0 0 1 1 1 1
  spline S275 degree 3 poles (24.5079, -18.6183) (25.255, -18.6183) (25.9932, -18.6183) (26.7404, -18.6183) knots 0 0 0 0 1 1 1 1
  spline S276 degree 3 poles (26.7404, -18.6183) (26.7404, -20.8812) (26.7404, -23.1456) (26.7404, -25.4191) knots 0 0 0 0 1 1 1 1
  spline S277 degree 3 poles (26.7404, -25.4191) (27.2141, -25.4191) (27.679, -25.4191) (28.1503, -25.4191) knots 0 0 0 0 1 1 1 1
  spline S278 degree 3 poles (28.1503, -25.4191) (28.1503, -26.8497) (28.1503, -28.2713) (28.1503, -29.7059) knots 0 0 0 0 1 1 1 1
  spline S279 degree 3 poles (28.1503, -29.7059) (27.4663, -29.7059) (26.7808, -29.7059) (26.0838, -29.7059) knots 0 0 0 0 1 1 1 1
  spline S280 degree 3 poles (11.2764, -29.1592) (11.2764, -29.3447) (11.2764, -29.5188) (11.2764, -29.6994) knots 0 0 0 0 1 1 1 1
  spline S281 degree 3 poles (11.2764, -29.6994) (9.5916, -29.6994) (7.9119, -29.6994) (6.2256, -29.6994) knots 0 0 0 0 1 1 1 1
  spline S282 degree 3 poles (6.2256, -29.6994) (6.2256, -28.2793) (6.2256, -26.8578) (6.2256, -25.4271) knots 0 0 0 0 1 1 1 1
  spline S283 degree 3 poles (6.2256, -25.4271) (6.6889, -25.4271) (7.1538, -25.4271) (7.6276, -25.4271) knots 0 0 0 0 1 1 1 1
  spline S284 degree 3 poles (7.6276, -25.4271) (7.6276, -23.1536) (7.6276, -20.8892) (7.6276, -18.6183) knots 0 0 0 0 1 1 1 1
  spline S285 degree 3 poles (7.6276, -18.6183) (8.3747, -18.6183) (9.1128, -18.6183) (9.86, -18.6183) knots 0 0 0 0 1 1 1 1
  spline S286 degree 3 poles (9.86, -18.6183) (9.86, -20.8813) (9.86, -23.1457) (9.86, -25.4192) knots 0 0 0 0 1 1 1 1
  spline S287 degree 3 poles (9.86, -25.4192) (10.3337, -25.4192) (10.7986, -25.4192) (11.2764, -25.4192) knots 0 0 0 0 1 1 1 1
  spline S288 degree 3 poles (11.2764, -25.4192) (11.2764, -26.6681) (11.2764, -27.908) (11.2764, -29.1592) knots 0 0 0 0 1 1 1 1
  spline S289 degree 3 poles (30.1388, -7.9504) (30.1388, -6.9221) (30.1388, -5.9051) (30.1388, -4.8791) knots 0 0 0 0 1 1 1 1
  spline S290 degree 3 poles (30.1388, -4.8791) (29.6691, -4.8791) (29.2042, -4.8791) (28.7329, -4.8791) knots 0 0 0 0 1 1 1 1
  spline S291 degree 3 poles (28.7329, -4.8791) (28.7329, -3.4484) (28.7329, -2.0269) (28.7329, -0.5988) knots 0 0 0 0 1 1 1 1
  spline S292 degree 3 poles (28.7329, -0.5988) (30.4112, -0.5988) (32.0909, -0.5988) (33.7771, -0.5988) knots 0 0 0 0 1 1 1 1
  spline S293 degree 3 poles (33.7771, -0.5988) (33.7771, -2.0189) (33.7771, -3.4404) (33.7771, -4.8711) knots 0 0 0 0 1 1 1 1
  spline S294 degree 3 poles (33.7771, -4.8711) (33.3139, -4.8711) (32.849, -4.8711) (32.3752, -4.8711) knots 0 0 0 0 1 1 1 1
  spline S295 degree 3 poles (32.3752, -4.8711) (32.3752, -7.1446) (32.3752, -9.409) (32.3752, -11.6799) knots 0 0 0 0 1 1 1 1
  spline S296 degree 3 poles (32.3752, -11.6799) (31.6281, -11.6799) (30.8899, -11.6799) (30.1388, -11.6799) knots 0 0 0 0 1 1 1 1
  spline S297 degree 3 poles (30.1388, -11.6799) (30.1388, -10.4415) (30.1388, -9.2017) (30.1388, -7.9504) knots 0 0 0 0 1 1 1 1
  spline S298 degree 3 poles (26.7445, -9.4312) (26.7445, -10.1862) (26.7445, -10.9298) (26.7445, -11.6799) knots 0 0 0 0 1 1 1 1
  spline S299 degree 3 poles (26.7445, -11.6799) (26.0013, -11.6799) (25.2631, -11.6799) (24.516, -11.6799) knots 0 0 0 0 1 1 1 1
  spline S300 degree 3 poles (24.516, -11.6799) (24.516, -9.417) (24.516, -7.1526) (24.516, -4.8791) knots 0 0 0 0 1 1 1 1
  spline S301 degree 3 poles (24.516, -4.8791) (24.0423, -4.8791) (23.5774, -4.8791) (23.1061, -4.8791) knots 0 0 0 0 1 1 1 1
  spline S302 degree 3 poles (23.1061, -4.8791) (23.1061, -3.4484) (23.1061, -2.0269) (23.1061, -0.5988) knots 0 0 0 0 1 1 1 1
  spline S303 degree 3 poles (23.1061, -0.5988) (24.7843, -0.5988) (26.4641, -0.5988) (28.1503, -0.5988) knots 0 0 0 0 1 1 1 1
  spline S304 degree 3 poles (28.1503, -0.5988) (28.1503, -2.0189) (28.1503, -3.4404) (28.1503, -4.8711) knots 0 0 0 0 1 1 1 1
  spline S305 degree 3 poles (28.1503, -4.8711) (27.6871, -4.8711) (27.2222, -4.8711) (26.7445, -4.8711) knots 0 0 0 0 1 1 1 1
  spline S306 degree 3 poles (26.7445, -4.8711) (26.7445, -6.3934) (26.7445, -7.9066) (26.7445, -9.4312) knots 0 0 0 0 1 1 1 1
  spline S307 degree 3 poles (31.2619, -17.0922) (30.7554, -17.6092) (30.1342, -17.8896) (29.4331, -17.9199) knots 0 0 0 0 1 1 1 1
  spline S308 degree 3 poles (29.4331, -17.9199) (28.5433, -17.9582) (27.6506, -17.9291) (26.7518, -17.9291) knots 0 0 0 0 1 1 1 1
  spline S309 degree 3 poles (26.7518, -17.9291) (26.7518, -16.0754) (26.7518, -14.2063) (26.7518, -12.3261) knots 0 0 0 0 1 1 1 1
  spline S310 degree 3 poles (26.7518, -12.3261) (26.7817, -12.3261) (26.8108, -12.3261) (26.8399, -12.3261) knots 0 0 0 0 1 1 1 1
  spline S311 degree 3 poles (26.8399, -12.3261) (27.5727, -12.3261) (28.3054, -12.3239) (29.0381, -12.3269) knots 0 0 0 0 1 1 1 1
  spline S312 degree 3 poles (29.0381, -12.3269) (29.5596, -12.329) (30.0644, -12.4183) (30.5351, -12.6532) knots 0 0 0 0 1 1 1 1
  spline S313 degree 3 poles (30.5351, -12.6532) (31.2249, -12.9974) (31.68, -13.5405) (31.8752, -14.2875) knots 0 0 0 0 1 1 1 1
  spline S314 degree 3 poles (31.8752, -14.2875) (32.0758, -15.0551) (32.0308, -15.8079) (31.6638, -16.5205) knots 0 0 0 0 1 1 1 1
  spline S315 degree 3 poles (31.6638, -16.5205) (31.5593, -16.7233) (31.401, -16.8984) (31.2619, -17.0922) knots 0 0 0 0 1 1 1 1
  spline S316 degree 3 poles (29.4325, -16.6445) (29.9645, -16.5062) (30.3086, -16.1687) (30.4751, -15.6498) knots 0 0 0 0 1 1 1 1
  spline S317 degree 3 poles (30.4751, -15.6498) (30.5647, -15.3705) (30.5663, -15.0838) (30.5242, -14.7949) knots 0 0 0 0 1 1 1 1
  spline S318 degree 3 poles (30.5242, -14.7949) (30.4264, -14.1244) (29.9248, -13.6453) (29.2473, -13.6029) knots 0 0 0 0 1 1 1 1
  spline S319 degree 3 poles (29.2473, -13.6029) (28.8922, -13.5806) (28.5349, -13.5912) (28.1786, -13.5876) knots 0 0 0 0 1 1 1 1
  spline S320 degree 3 poles (28.1786, -13.5876) (28.1729, -13.5875) (28.167, -13.5963) (28.1623, -13.6001) knots 0 0 0 0 1 1 1 1
  spline S321 degree 3 poles (28.1623, -13.6001) (28.1623, -14.6276) (28.1623, -15.6542) (28.1623, -16.7091) knots 0 0 0 0 1 1 1 1
  spline S322 degree 3 poles (28.1623, -16.7091) (28.5839, -16.6888) (28.9989, -16.6687) (29.4325, -16.6445) knots 0 0 0 0 1 1 1 1
  spline S323 degree 3 poles (25.0631, -12.7063) (26.0221, -13.4204) (26.0292, -15.3556) (24.6542, -15.8845) knots 0 0 0 0 1 1 1 1
  spline S324 degree 3 poles (24.6542, -15.8845) (25.0223, -16.5698) (25.39, -17.2541) (25.7624, -17.9475) knots 0 0 0 0 1 1 1 1
  spline S325 degree 3 poles (25.7624, -17.9475) (25.2172, -17.9475) (24.6869, -17.9475) (24.1535, -17.9475) knots 0 0 0 0 1 1 1 1
  spline S326 degree 3 poles (24.1535, -17.9475) (23.866, -17.3431) (23.5772, -16.739) (23.2923, -16.1331) knots 0 0 0 0 1 1 1 1
  spline S327 degree 3 poles (23.2923, -16.1331) (23.2595, -16.0634) (23.2246, -16.0322) (23.1426, -16.0352) knots 0 0 0 0 1 1 1 1
  spline S328 degree 3 poles (23.1426, -16.0352) (22.9424, -16.0425) (22.7418, -16.0376) (22.5324, -16.0376) knots 0 0 0 0 1 1 1 1
  spline S329 degree 3 poles (22.5324, -16.0376) (22.5324, -16.6761) (22.5324, -17.308) (22.5324, -17.9455) knots 0 0 0 0 1 1 1 1
  spline S330 degree 3 poles (22.5324, -17.9455) (22.0586, -17.9455) (21.5938, -17.9455) (21.1233, -17.9455) knots 0 0 0 0 1 1 1 1
  spline S331 degree 3 poles (21.1233, -17.9455) (21.1233, -16.0751) (21.1233, -14.2057) (21.1233, -12.3284) knots 0 0 0 0 1 1 1 1
  spline S332 degree 3 poles (21.1233, -12.3284) (21.1523, -12.327) (21.1813, -12.3245) (21.2104, -12.3245) knots 0 0 0 0 1 1 1 1
  spline S333 degree 3 poles (21.2104, -12.3245) (22.0835, -12.3243) (22.9565, -12.3226) (23.8296, -12.325) knots 0 0 0 0 1 1 1 1
  spline S334 degree 3 poles (23.8296, -12.325) (24.2757, -12.3262) (24.6935, -12.4266) (25.0631, -12.7063) knots 0 0 0 0 1 1 1 1
  spline S335 degree 3 poles (23.9814, -14.7249) (24.2534, -14.5657) (24.3663, -14.2948) (24.2836, -13.9997) knots 0 0 0 0 1 1 1 1
  spline S336 degree 3 poles (24.2836, -13.9997) (24.2146, -13.754) (23.9952, -13.5694) (23.7247, -13.5566) knots 0 0 0 0 1 1 1 1
  spline S337 degree 3 poles (23.7247, -13.5566) (23.437, -13.543) (23.1484, -13.549) (22.8603, -13.547) knots 0 0 0 0 1 1 1 1
  spline S338 degree 3 poles (22.8603, -13.547) (22.7521, -13.5462) (22.6439, -13.5469) (22.5377, -13.5469) knots 0 0 0 0 1 1 1 1
  spline S339 degree 3 poles (22.5377, -13.5469) (22.5377, -13.9753) (22.5377, -14.3901) (22.5377, -14.8074) knots 0 0 0 0 1 1 1 1
  spline S340 degree 3 poles (22.5377, -14.8074) (22.9018, -14.8074) (23.2583, -14.8134) (23.6144, -14.804) knots 0 0 0 0 1 1 1 1
  spline S341 degree 3 poles (23.6144, -14.804) (23.7324, -14.8009) (23.8494, -14.7585) (23.9814, -14.7249) knots 0 0 0 0 1 1 1 1
  spline S342 degree 3 poles (16.1445, -17.8902) (15.0088, -17.4609) (14.4002, -16.6354) (14.2807, -15.4476) knots 0 0 0 0 1 1 1 1
  spline S343 degree 3 poles (14.2807, -15.4476) (14.2022, -14.6676) (14.3755, -13.9444) (14.8619, -13.3182) knots 0 0 0 0 1 1 1 1
  spline S344 degree 3 poles (14.8619, -13.3182) (15.3695, -12.6649) (16.0569, -12.3333) (16.8716, -12.2536) knots 0 0 0 0 1 1 1 1
  spline S345 degree 3 poles (16.8716, -12.2536) (17.5266, -12.1895) (18.1513, -12.2977) (18.7243, -12.6285) knots 0 0 0 0 1 1 1 1
  spline S346 degree 3 poles (18.7243, -12.6285) (19.4853, -13.068) (19.9233, -13.7403) (20.0663, -14.5989) knots 0 0 0 0 1 1 1 1
  spline S347 degree 3 poles (20.0663, -14.5989) (20.1938, -15.3643) (20.0864, -16.0975) (19.6675, -16.7638) knots 0 0 0 0 1 1 1 1
  spline S348 degree 3 poles (19.6675, -16.7638) (19.2139, -17.4852) (18.5444, -17.8837) (17.713, -18.02) knots 0 0 0 0 1 1 1 1
  spline S349 degree 3 poles (17.713, -18.02) (17.1838, -18.1067) (16.6625, -18.0645) (16.1445, -17.8902) knots 0 0 0 0 1 1 1 1
  spline S350 degree 3 poles (17.4159, -16.7667) (17.7911, -16.7171) (18.101, -16.5451) (18.3279, -16.2445) knots 0 0 0 0 1 1 1 1
  spline S351 degree 3 poles (18.3279, -16.2445) (18.7026, -15.748) (18.7615, -15.1877) (18.6061, -14.6024) knots 0 0 0 0 1 1 1 1
  spline S352 degree 3 poles (18.6061, -14.6024) (18.437, -13.9655) (17.929, -13.5557) (17.2886, -13.5143) knots 0 0 0 0 1 1 1 1
  spline S353 degree 3 poles (17.2886, -13.5143) (16.6486, -13.473) (16.0963, -13.806) (15.8437, -14.393) knots 0 0 0 0 1 1 1 1
  spline S354 degree 3 poles (15.8437, -14.393) (15.6748, -14.7855) (15.6525, -15.194) (15.7459, -15.6076) knots 0 0 0 0 1 1 1 1
  spline S355 degree 3 poles (15.7459, -15.6076) (15.9245, -16.3984) (16.6257, -16.8897) (17.4159, -16.7667) knots 0 0 0 0 1 1 1 1
  spline S356 degree 3 poles (10.6386, -14.4201) (10.9986, -14.4201) (11.3473, -14.4201) (11.7049, -14.4201) knots 0 0 0 0 1 1 1 1
  spline S357 degree 3 poles (11.7049, -14.4201) (11.7049, -13.7229) (11.7049, -13.0303) (11.7049, -12.3311) knots 0 0 0 0 1 1 1 1
  spline S358 degree 3 poles (11.7049, -12.3311) (12.1785, -12.3311) (12.6432, -12.3311) (13.1148, -12.3311) knots 0 0 0 0 1 1 1 1
  spline S359 degree 3 poles (13.1148, -12.3311) (13.1148, -14.198) (13.1148, -16.0672) (13.1148, -17.9437) knots 0 0 0 0 1 1 1 1
  spline S360 degree 3 poles (13.1148, -17.9437) (12.6537, -17.9437) (12.1889, -17.9437) (11.712, -17.9437) knots 0 0 0 0 1 1 1 1
  spline S361 degree 3 poles (11.712, -17.9437) (11.712, -17.1955) (11.712, -16.4429) (11.712, -15.6849) knots 0 0 0 0 1 1 1 1
  spline S362 degree 3 poles (11.712, -15.6849) (10.9543, -15.6849) (10.2088, -15.6849) (9.4552, -15.6849) knots 0 0 0 0 1 1 1 1
  spline S363 degree 3 poles (9.4552, -15.6849) (9.4552, -16.4402) (9.4552, -17.1901) (9.4552, -17.9455) knots 0 0 0 0 1 1 1 1
  spline S364 degree 3 poles (9.4552, -17.9455) (8.9824, -17.9455) (8.5177, -17.9455) (8.0472, -17.9455) knots 0 0 0 0 1 1 1 1
  spline S365 degree 3 poles (8.0472, -17.9455) (8.0472, -16.0752) (8.0472, -14.206) (8.0472, -12.3306) knots 0 0 0 0 1 1 1 1
  spline S366 degree 3 poles (8.0472, -12.3306) (8.5119, -12.3306) (8.9766, -12.3306) (9.4503, -12.3306) knots 0 0 0 0 1 1 1 1
  spline S367 degree 3 poles (9.4503, -12.3306) (9.4503, -13.0222) (9.4503, -13.7148) (9.4503, -14.4201) knots 0 0 0 0 1 1 1 1
  spline S368 degree 3 poles (9.4503, -14.4201) (9.8484, -14.4201) (10.2378, -14.4201) (10.6386, -14.4201) knots 0 0 0 0 1 1 1 1
  spline S369 degree 3 poles (35.4182, -18.0602) (34.6784, -18.0797) (33.9769, -17.9731) (33.3454, -17.5812) knots 0 0 0 0 1 1 1 1
  spline S370 degree 3 poles (33.3454, -17.5812) (33.1571, -17.4644) (32.9868, -17.3185) (32.8062, -17.1844) knots 0 0 0 0 1 1 1 1
  spline S371 degree 3 poles (32.8062, -17.1844) (33.0667, -16.8029) (33.312, -16.4435) (33.5594, -16.0811) knots 0 0 0 0 1 1 1 1
  spline S372 degree 3 poles (33.5594, -16.0811) (33.9548, -16.4754) (34.416, -16.7195) (34.9593, -16.8) knots 0 0 0 0 1 1 1 1
  spline S373 degree 3 poles (34.9593, -16.8) (35.1855, -16.8335) (35.4142, -16.8493) (35.6367, -16.784) knots 0 0 0 0 1 1 1 1
  spline S374 degree 3 poles (35.6367, -16.784) (35.7366, -16.7547) (35.8382, -16.7105) (35.9212, -16.649) knots 0 0 0 0 1 1 1 1
  spline S375 degree 3 poles (35.9212, -16.649) (36.1534, -16.4769) (36.1425, -16.1803) (35.9019, -16.0198) knots 0 0 0 0 1 1 1 1
  spline S376 degree 3 poles (35.9019, -16.0198) (35.6796, -15.8714) (35.4179, -15.8315) (35.1656, -15.765) knots 0 0 0 0 1 1 1 1
  spline S377 degree 3 poles (35.1656, -15.765) (34.7748, -15.6619) (34.3771, -15.5761) (33.9981, -15.4393) knots 0 0 0 0 1 1 1 1
  spline S378 degree 3 poles (33.9981, -15.4393) (33.5664, -15.2834) (33.2291, -15.0004) (33.074, -14.5448) knots 0 0 0 0 1 1 1 1
  spline S379 degree 3 poles (33.074, -14.5448) (32.7844, -13.6938) (33.2042, -12.8062) (34.0699, -12.4405) knots 0 0 0 0 1 1 1 1
  spline S380 degree 3 poles (34.0699, -12.4405) (34.4539, -12.2782) (34.8576, -12.223) (35.2711, -12.2358) knots 0 0 0 0 1 1 1 1
  spline S381 degree 3 poles (35.2711, -12.2358) (35.9773, -12.2575) (36.6315, -12.4423) (37.2046, -12.8709) knots 0 0 0 0 1 1 1 1
  spline S382 degree 3 poles (37.2046, -12.8709) (37.2652, -12.9163) (37.3229, -12.9656) (37.3871, -13.0172) knots 0 0 0 0 1 1 1 1
  spline S383 degree 3 poles (37.3871, -13.0172) (37.1302, -13.3644) (36.8759, -13.7079) (36.6186, -14.0557) knots 0 0 0 0 1 1 1 1
  spline S384 degree 3 poles (36.6186, -14.0557) (36.2925, -13.7907) (35.9294, -13.6098) (35.5216, -13.5236) knots 0 0 0 0 1 1 1 1
  spline S385 degree 3 poles (35.5216, -13.5236) (35.2713, -13.4707) (35.019, -13.4418) (34.7671, -13.5119) knots 0 0 0 0 1 1 1 1
  spline S386 degree 3 poles (34.7671, -13.5119) (34.7061, -13.5289) (34.6447, -13.5556) (34.5927, -13.5913) knots 0 0 0 0 1 1 1 1